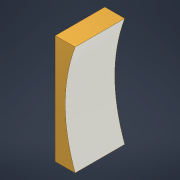
# Autodesk Inventor part: LED Reflector
Saved by Autodesk Inventor 2022 (Build 260153000, 153)
## iProperties
Created: 2021-08-06
Part Number: LED Reflector
Material: Generic
Document SubType Name: Modeling
Designer: sidsa
Density: 1 g/cm^3
Appearance: Brass - Satin
Author: sidsa
Autodesk Inventor part; units mm, degrees
ref_plane "YZ Plane" through (0, 0, 0) normal (1, 0, 0) x (0, 1, 0)
ref_plane "XZ Plane" through (0, 0, 0) normal (0, 1, 0) x (-1, 0, 0)
ref_plane "XY Plane" through (0, 0, 0) normal (0, 0, 1) x (1, 0, 0)
ref_plane "Work Plane1" through (6.35, -34.925, 15.875) normal (0, 0, 1) x (1, 0, 0)
sketch "Sketch3" plane through (6.35, -34.925, 15.875) normal (0, 0, 1) x (1, 0, 0)
  line L0 (1.5875, 69.85) -> (1.5875, 0) projected
  line L1 (14.2875, 0) -> (1.5875, 34.925) construction
  line L2 (1.5875, 34.925) -> (14.2875, 69.85) construction
  spline S0 degree 2 poles (14.2875, 0) (1.5875, 34.925) (14.2875, 69.85) knots 1 1 1 2 2 2
  line L3 (1.5875, 69.85) -> (14.2875, 69.85)
  line L4 (14.2875, 0) -> (1.5875, 0)
  point P0 (-6.35, 34.925)
  dimension "d9" = 12.7
  dimension "d10" = 12.7
  constraints: 4 end point, 1 midpoint, 1 parallel, 4 other
  measures "d9" distance of L0.start L2.end
  measures "d10" distance of L0.end L1.start
extrude "Extrusion3" add sketch "Sketch3" against normal blind 31.75
body "Solid1"
